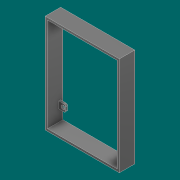
# Autodesk Inventor part: struttura
Saved by Autodesk Inventor 2020 (Build 240168000, 168)
## iProperties
Created: 2025-02-23
Part Number: struttura
Material: Plastica ABS
Document SubType Name: Modeling
Designer: Nicola Milia
Density: 1.06 g/cm^3
Appearance: Liscia - Bianco
Author: Nicola Milia
## iProperties of the stored document _Stampa 3D.ipt
Created: 2025-02-23
Part Number: _Stampa 3D
Material: Generico
Document SubType Name: Modeling
Designer: Nicola Milia
Density: 1 g/cm^3
Appearance: Default
Author: Nicola Milia
Autodesk Inventor part; units mm, degrees
ref_plane "YZ Plane" through (0, 0, 0) normal (1, 0, 0) x (0, 1, 0)
ref_plane "XZ Plane" through (0, 0, 0) normal (0, 1, 0) x (-1, 0, 0)
ref_plane "Piano di lavoro1" through (0, 0, 0) normal (0, 0, 1) x (1, 0, 0)
sketch "Schizzo1" plane through (0, 0, 0) normal (0, 0, 1) x (1, 0, 0)
  line L0 (42, 54.3) -> (-33, 54.3) projected
  line L1 (42, 19.3) -> (42, 54.3) projected
  line L2 (-45, -61) -> (45, -61) projected
  line L3 (-45, 61) -> (-45, -61) projected
  line L4 (45, 61) -> (-45, 61) projected
  circle A0 centre (-40, 57.5) radius 2.5 projected
  circle A1 centre (-40, -42) radius 2.5 projected
  circle A2 centre (41.5, -42) radius 2.5 projected
  circle A3 centre (41.5, 57.5) radius 2.5 projected
  line L5 (45, -61) -> (45, 61) projected
  line L6 (-45.5, 61.5) -> (-45.5, -61.5)
  line L7 (-45.5, -61.5) -> (45.5, -61.5)
  line L8 (45.5, -61.5) -> (45.5, 61.5)
  line L9 (45.5, 61.5) -> (-45.5, 61.5)
  line L10 (48.5, 64.5) -> (48.5, -64.5)
  line L11 (48.5, -64.5) -> (-48.5, -64.5)
  line L12 (-48.5, -64.5) -> (-48.5, 64.5)
  line L13 (-48.5, 64.5) -> (48.5, 64.5)
  point P0 (0, 0)
  dimension "d0" = 0.5
  dimension "d1" = 3
  constraints: 16 end point, 6 other
  measures "d0" distance between parallel lines of L4 L9
  measures "d1" distance between parallel lines of L8 L10
extrude "Estrusione1" add sketch "Schizzo1" along normal blind 17.25 contours L10 L11 L12 L13
move faces "Sposta1" translate (0, 0, -3) faces at (-47.5, 20.5, 0)
sketch "Schizzo2" plane through (0, 0, 0) normal (0, 0, 1) x (1, 0, 0)
  circle A0 centre (41.5, 57.5) radius 2.5 projected
  circle A1 centre (-40, 57.5) radius 2.5 projected
  circle A2 centre (41.5, -42) radius 2.5 projected
  circle A3 centre (-40, -42) radius 2.5 projected
  line L0 (-45.5, 61.5) -> (45.5, 61.5) projected
  line L1 (-45.5, 61.5) -> (45.5, 61.5) projected
  line L2 (45.5, 61.5) -> (45.5, -61.5) projected
  line L3 (45.5, 61.5) -> (45.5, -61.5) projected
  line L4 (-45.5, -61.5) -> (-45.5, 61.5) projected
  line L5 (-45.5, -61.5) -> (-45.5, 61.5) projected
  line L6 (45.5, -61.5) -> (-45.5, -61.5) projected
  line L7 (45.5, -61.5) -> (-45.5, -61.5) projected
  line L8 (45.5, 61.5) -> (37.5, 61.5)
  line L9 (37.5, 61.5) -> (37.5, 55.5)
  line L10 (39.5, 53.5) -> (45.5, 53.5)
  line L11 (45.5, 53.5) -> (45.5, 61.5)
  arc A4 (37.5, 55.5) -> (39.5, 53.5) centre (39.5, 55.5) ccw
  line L12 (-45.5, 61.5) -> (-35.5, 61.5)
  line L13 (-35.5, 61.5) -> (-35.5, 53.5)
  line L14 (-37.5, 51.5) -> (-45.5, 51.5)
  line L15 (-45.5, 51.5) -> (-45.5, 61.5)
  arc A5 (-37.5, 51.5) -> (-35.5, 53.5) centre (-37.5, 53.5) ccw
  line L16 (-45.5, -61.5) -> (-45.5, 61.5) projected
  line L17 (-45.5, -37.8875) -> (-45.5, -46.8794)
  line L18 (-45.5, -46.496) -> (-38.5282, -46.496)
  line L19 (-36.5282, -44.496) -> (-36.5282, -39.504)
  line L20 (-38.5282, -37.504) -> (-45.5, -37.504)
  arc A6 (-38.5282, -46.496) -> (-36.5282, -44.496) centre (-38.5282, -44.496) ccw
  arc A7 (-36.5282, -39.504) -> (-38.5282, -37.504) centre (-38.5282, -39.504) ccw
  line L21 (45.5, 61.5) -> (45.5, -61.5) projected
  line L22 (45.5, -45.9102) -> (45.5, -38.0898)
  line L23 (45.5, -38.0898) -> (40.1, -38.0898)
  line L24 (38.1, -40.0898) -> (38.1, -43.9102)
  line L25 (40.1, -45.9102) -> (45.5, -45.9102)
  arc A8 (38.1, -43.9102) -> (40.1, -45.9102) centre (40.1, -43.9102) ccw
  arc A9 (40.1, -38.0898) -> (38.1, -40.0898) centre (40.1, -40.0898) ccw
  point P0 (0, 0)
  point P1 (37.5, 53.5)
  point P2 (-35.5, 51.5)
  point P3 (-36.5282, -42.3835)
  point P4 (-36.5282, -42)
  point P5 (38.1, -38.0898)
  dimension "d7" = 8
  dimension "d8" = 8
  dimension "d9" = 2
  dimension "d10" = 10
  dimension "d11" = 10
  dimension "d12" = 2
  dimension "d13" = 2
  dimension "d14" = 7.4
  dimension "d15" = 2
  constraints: 32 end point, 12 point on circle, 12 tangent, 8 parallel, 7 point on line, 6 centre point, 4 perpendicular, 2 equal radius, 2 horizontal, 3 other
  measures "d7" distance of L10.end point (37.5, 53.5)
  measures "d8" distance of point (37.5, 53.5) L8.end
  measures "d9" radius of A4
  measures "d10" distance of point (-35.5, 51.5) L14.end
  measures "d11" distance of L12.end point (-35.5, 51.5)
  measures "d12" radius of A5
  measures "d13" radius of A6
  measures "d14" distance of point (38.1, -38.09) L22.end
  measures "d15" radius of A8
extrude "Estrusione2" add sketch "Schizzo2" along normal blind 2.5 contours L0 L13 A5 L14 L4 | L0 L2 L10 A4 L9 | L20 A7 L19 A6 L18 L4 | L2 L25 A8 L24 A9 L23
